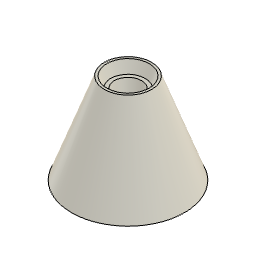
Step1-Cone_Support-4X (Autodesk Fusion 360 design; units mm, degrees)
Autodesk Fusion 360 part; units mm, degrees
sketch "Sketch1" plane through (0, 0, 0) normal (0, 0, 1) x (1, 0, 0)
  circle A0 centre (0, 0) radius 12.5
  dimension "d1" = 25
  constraint coincident A0.centre origin
  measures "d1" diameter of A0
extrude "Extrude1" add sketch "Sketch1" along normal blind 50 draft -20
ref_plane "WorkPlane1" through (0, 0, 20) normal (0, 0, -1) x (-1, 0, 0)
sketch "Sketch2" plane through (0, 0, 20) normal (0, 0, -1) x (1, 0, 0)
  line L0 (-29.1511, -26.6162) -> (43.8534, -26.6162)
  line L1 (43.8534, -26.6162) -> (43.8534, 28.6441)
  line L2 (43.8534, 28.6441) -> (-29.1511, 28.6441)
  line L3 (-29.1511, 28.6441) -> (-29.1511, -26.6162)
  constraint horizontal L0
  constraint vertical L1
  constraint horizontal L2
  constraint vertical L3
extrude "Extrude2" cut sketch "Sketch2" against normal blind 30
ref_plane "WorkPlane2" through (0, 0, 20) normal (0, 0, 1) x (-1, 0, 0)
sketch "Sketch3" plane through (0, 0, 20) normal (0, 0, 1) x (1, 0, 0)
  circle A0 centre (0, 0) radius 3
  circle A1 centre (0, 0) radius 4.7
  dimension "d8" = 6
  dimension "d9" = 9.4
  constraint coincident A0.centre A1.centre
  constraint concentric A0 A1
  measures "d8" diameter of A0
  measures "d9" diameter of A1
extrude "Extrude4" cut sketch "Sketch3" against normal blind 30 contours A0
extrude "Extrude3" cut sketch "Sketch3" against normal blind 2.4 draft -20 contours A0 | A1
